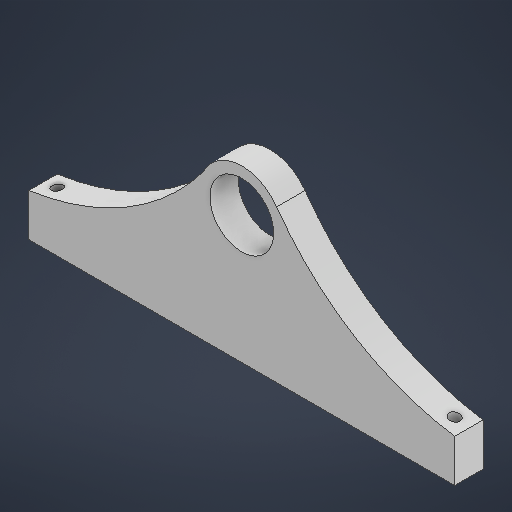
# Autodesk Inventor part: podstawa
Saved by Autodesk Inventor 2026.2 (Build 302298000, 298)
## iProperties
Created: 2025-11-25
Part Number: podstawa
Material: Generic
Document SubType Name: Modeling
Designer: janek
Density: 1 g/cm^3
Appearance: Default
Author: janek
Autodesk Inventor part; units mm, degrees
ref_plane "YZ Plane" through (0, 0, 0) normal (1, 0, 0) x (0, 1, 0)
ref_plane "XZ Plane" through (0, 0, 0) normal (0, 1, 0) x (-1, 0, 0)
ref_plane "XY Plane" through (0, 0, 0) normal (0, 0, 1) x (1, 0, 0)
sketch "Sketch1" plane through (0, 0, 0) normal (0, 0, 1) x (1, 0, 0)
  line L0 (0, 0) -> (120, 0)
  line L1 (120, 0) -> (120, 12)
  line L2 (120, 12) -> (0, 12)
  line L3 (0, 12) -> (0, 0)
  line L4 (48, 12) -> (72, 12)
  line L5 (72, 12) -> (72, 36)
  line L6 (72, 36) -> (48, 36)
  line L7 (48, 36) -> (48, 12)
  circle A0 centre (60, 36) radius 12
  arc A1 (0, 12) -> (49.1767, 41.1822) centre (-10.4643, 85.6604) ccw
  arc A2 (69.8235, 42.892) -> (120, 12) centre (130.7289, 85.6223) ccw
  circle A3 centre (60, 36) radius 9
  point P0 (120, 6)
  point P1 (0, 6)
  dimension "d30" = 120
  dimension "d31" = 18
  dimension "d32" = 74.4
  dimension "d33" = 74.4
  dimension "d34" = 24
  dimension "d35" = 24
  dimension "d36" = 73.6604
  dimension "d37" = 12
  dimension "d38" = 30.892
  constraints: 16 end point, 7 point on circle, 4 centre point, 4 parallel, 3 midpoint, 2 horizontal, 2 perpendicular, 1 coincident, 1 point on line, 1 tangent
  measures "d30" distance of L1.end L2.end
  measures "d31" diameter of A3
  measures "d32" radius of A2
  measures "d33" radius of A1
  measures "d34" diameter of A0
  measures "d35" distance of L6.end L4.start
  measures "d36" distance from line of L2 A1.centre
  measures "d37" distance between parallel lines of L0 L2
  measures "d38" distance from line of L2 A2.start
extrude "Extrusion1" add sketch "Sketch1" along normal blind 8 contours L3 L2 L1 L0 | A1 A0 L7 L2 | L2 L5 A0 A2 | L7 A0 L5 L2 | A0 L6 A3 | L6 A3 A0
sketch "Sketch2" plane through (0, 0, 0) normal (0, -1, 0) x (1, 0, 0)
  line L0 (0, 8) -> (120, 8) projected
  line L1 (0, 0) -> (0, 8) projected
  line L2 (120, 0) -> (120, 8) projected
  point P0 (4, 4)
  point P1 (116, 4)
  point P2 (120, 4)
  dimension "d12" = 4
  dimension "d13" = 4
  dimension "d14" = 4
  dimension "d15" = 4
  constraints: 1 midpoint
  measures "d12" distance from line of L0 point (4, 4)
  measures "d13" distance from line of L1 point (4, 4)
  measures "d14" distance of point (120, 4) point (116, 4)
  measures "d15" distance from line of L0 point (116, 4)
hole "Hole2" at (4, 0, 4) at (116, 0, 4) direction (0, 1, 0) diameter 3 end through all
body "Solid1"
